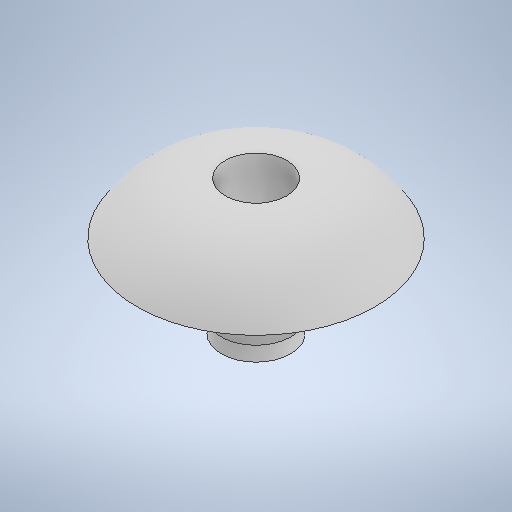
# Autodesk Inventor part: Water Sensor Bouy 3
Saved by Autodesk Inventor 2025 (Build 290162000, 162)
## iProperties
Created: 2024-06-24
Part Number: Water Sensor Bouy 3
Material: Generic
Document SubType Name: Modeling
Designer: track
Density: 1 g/cm^3
Appearance: Default
Mass: 131.013 g
Surface Area: 2370.25 cm^2
Volume: 131.013 cm^3
Author: track
## iProperties of the stored document Water Sensor Bouy 3_3DPrint.ipt
Created: 2024-06-24
Part Number: Water Sensor Bouy 3_3DPrint
Material: Generic
Document SubType Name: Modeling
Designer: track
Density: 1 g/cm^3
Appearance: Default
Author: track
Autodesk Inventor part; units mm, degrees
ref_plane "YZ Plane" through (0, 0, 0) normal (1, 0, 0) x (0, 1, 0)
ref_plane "XZ Plane" through (0, 0, 0) normal (0, 1, 0) x (-1, 0, 0)
sketch "Sketch2" plane through (0, 0, 0) normal (0, 0, 1) x (1, 0, 0)
  line L0 (0, 0) -> (0, 152.4)
  line L1 (30.98, 2.0961) -> (30.98, 101.6)
  arc A0 (119.88, 74.5869) -> (32.1414, 1.741) centre (200.5975, -111.8935) ccw
  arc A1 (30.98, 2.0961) -> (32.1414, 1.741) centre (31.615, 2.0961) ccw
  line L2 (30.98, 101.6) -> (30.98, 127)
  arc A2 (119.88, 74.5869) -> (30.98, 127) centre (30.98, 25.4) ccw
  line L3 (30.98, 127) -> (25.9, 127)
  line L4 (31.98, 125.995) -> (31.98, 101.6)
  line L5 (31.98, 101.6) -> (31.98, 3.2837)
  arc A3 (118.4675, 75.0619) -> (31.98, 3.2837) centre (200.5975, -111.8935) ccw
  arc A4 (118.4675, 75.0619) -> (31.98, 125.995) centre (30.98, 25.4) ccw
  point P0 (30.98, 0)
  point P1 (43.68, 0)
  point P2 (114.9367, 72.3685)
  dimension "d0" = 30.98
  dimension "d1" = 101.6
  dimension "d2" = 152.4
  dimension "d76" = 88.9
  dimension "d77" = 203.2
  dimension "d80" = 0.635
  dimension "d91" = 25.4
  dimension "d92" = 101.6
  dimension "d93" = 88.9
  dimension "d94" = 5.08
  dimension "d95" = 0
  dimension "d96" = 1
  constraints: 12 end point, 12 point on circle, 5 centre point, 3 tangent, 3 vertical, 1 horizontal, 1 point on line, 3 other
  measures "d0" distance between parallel lines of L0 L1
  measures "d1" distance of point (30.98, 0) L1.end
  measures "d2" distance of L0.start L0.end
  measures "d76" distance of L1.end point (114.937, 72.368)
  measures "d77" radius of A0
  measures "d80" radius of A1
  measures "d91" distance of L1.end L2.end
  measures "d92" radius of A2
  measures "d93" distance from line of L1 A0.start
  measures "d94" distance of L2.end L3.end
  measures "d95" vertical distance of L0.start point (30.98, 0)
  measures "d96" distance between parallel lines of L2 L4
revolve "Revolution1" add sketch "Sketch2" angle 360 about axis through (0, 0, 0) along (0, 1, 0)
ref_plane "Work Plane1" through (0, -111.8935, 0) normal (0, 1, 0) x (-1, 0, 0)
sketch "Sketch4" plane through (0, -111.8935, 0) normal (0, 1, 0) x (-1, 0, 0)
  circle A0 centre (0, 88.9) radius 3
  line L0 (0, 0) -> (0, 115.8951)
  dimension "d19" = 6
  dimension "d20" = 88.9
  constraints: 2 coincident, 2 end point, 1 centre point, 1 point on line, 1 vertical
  measures "d19" diameter of A0
  measures "d20" distance of point (0, 0) A0.centre
extrude "Extrusion1" cut sketch "Sketch4" along normal blind 173.0375
pattern_circular "Circular Pattern1" count 3 over 360 about axis through (0, 64.5481, 0) along (0, 1, 0) of "Extrusion1"
sketch "Sketch11" plane through (0, 0, 0) normal (0, 1, 0) x (-1, 0, 0)
  circle A0 centre (0, 0) radius 34.98
  circle A1 centre (0, 0) radius 30.98
  circle A2 centre (0, 0) radius 30.98 projected
  dimension "d83" = 0
  dimension "d84" = 4
  constraints: 2 centre point, 2 coincident
  measures "d83" radial gap between concentric circles of A2 A1
  measures "d84" radial gap between concentric circles of A1 A0
extrude "Extrusion7" add sketch "Sketch11" along normal blind 12.7 and the other way blind 8.89
ref_plane "Work Plane3" through (0, 0, -34.98) normal (0, 0, 1) x (1, 0, 0)
sketch "Sketch12" plane through (0, 0, -34.98) normal (0, 0, 1) x (1, 0, 0)
  line L0 (4.54, 0) -> (2.54, 0)
  line L1 (2.54, 0) -> (2.54, -8.89)
  line L2 (2.54, -8.89) -> (4.54, -8.89)
  line L3 (4.54, -8.89) -> (4.54, 0)
  line L4 (-2.54, 0) -> (-4.54, 0)
  line L5 (-4.54, 0) -> (-4.54, -8.89)
  line L6 (-4.54, -8.89) -> (-2.54, -8.89)
  line L7 (-2.54, -8.89) -> (-2.54, 0)
  line L8 (0, -8.89) -> (0, 0)
  line L9 (-34.98, -8.89) -> (34.98, -8.89) projected
  dimension "d56" = 8.89
  dimension "d57" = 2
  dimension "d58" = 2.54
  dimension "d85" = 0
  constraints: 18 end point, 4 parallel, 2 horizontal, 2 perpendicular, 2 point on line, 1 vertical, 2 other
  measures "d56" distance of L6.end L4.start
  measures "d57" distance of L0.start L0.end
  measures "d58" distance between parallel lines of L8 L1
  measures "d85" distance between parallel lines of L9 L6
extrude "Extrusion8" add sketch "Sketch12" along normal blind 1.27 and the other way blind 8.89
sketch "Sketch13" plane through (0, 0, -34.98) normal (0, 0, 1) x (1, 0, 0)
  line L0 (2.54, 0) -> (2.54, -8.89) projected
  line L1 (-2.54, -8.89) -> (2.54, -8.89) projected
  line L2 (2.54, 0) -> (-2.54, 0)
  line L3 (-2.54, 0) -> (-2.54, -8.89)
  line L4 (-2.54, -8.89) -> (2.54, -8.89)
  line L5 (2.54, -8.89) -> (2.54, 0)
  point P0 (0, 0)
  constraints: 8 end point, 2 parallel, 1 horizontal, 1 perpendicular
extrude "Extrusion9" cut sketch "Sketch13" along normal up to surface round surface about axis through (0, 64.5481, 0) along (0, 1, 0) radius 30.98 far side no
sketch "Sketch15" plane through (0, 0, -43.87) normal (0, 0, -1) x (-1, 0, 0)
  line L0 (2.54, -8.89) -> (2.54, 0) projected
  line L1 (34.98, -8.89) -> (34.98, 5.8397) projected
  line L2 (2.54, 0) -> (34.98, 0)
  line L3 (34.98, 0) -> (34.98, -2)
  line L4 (34.98, -2) -> (2.54, -2)
  line L5 (2.54, -2) -> (2.54, 0)
  point P0 (0, 0)
  dimension "d89" = 2
  constraints: 8 end point, 2 parallel, 1 horizontal, 1 perpendicular, 1 point on line
  measures "d89" distance between parallel lines of L4 L2
extrude "Extrusion10" cut sketch "Sketch15" against normal blind 63.5
sketch "Sketch16" plane through (-4.54, 0, -43.87) normal (-1, 0, 0) x (0, 0, 1)
  line L0 (2.54, -8.89) -> (2.54, 0)
  line L1 (0, -8.89) -> (0, 0) projected
  circle A0 centre (2.54, -3.81) radius 1.27
  circle A1 centre (2.54, -6.985) radius 1.27
  line L2 (9.1859, 0) -> (0, 0) projected
  line L3 (0, -8.89) -> (9.1859, -8.89) projected
  point P0 (43.87, 0)
  dimension "d68" = 2.54
  dimension "d69" = 2.54
  dimension "d70" = 2.54
  dimension "d71" = 3.81
  dimension "d90" = 1.905
  constraints: 2 centre point, 2 end point, 2 point on line, 1 vertical
  measures "d68" distance between parallel lines of L1 L0
  measures "d69" diameter of A1
  measures "d70" diameter of A0
  measures "d71" distance from line of L2 A0.centre
  measures "d90" distance from line of L3 A1.centre
extrude "Extrusion11" cut sketch "Sketch16" against normal up to surface (9.08 mm away) contours A1 L0 | L0 A1 | A0 L0 | L0 A0
body "Solid1"
